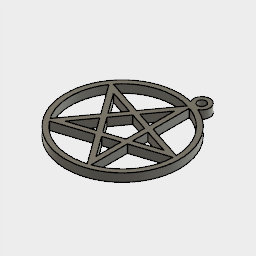
FPROJ_9_LIUYH (Autodesk Fusion 360 design; units mm, degrees)
Autodesk Fusion 360 part; units mm, degrees
sketch "草图1" plane through (0, 0, 0) normal (0, 1, 0) x (1, 0, 0)
  circle A0 centre (-5, 0) radius 34.7082
  arc A1 (-31.2161, 17.8361) -> (-30.0644, 19.4213) centre (-5, 0) ccw
  circle A2 centre (-65, 20) radius 2.5
  circle A3 centre (-65, 20) radius 4
  line L0 (-18.2574, 0) -> (-31.2161, -17.8361)
  line L1 (3.862, -30.4446) -> (-16.4033, -2.552)
  line L2 (-18.2574, 0) -> (-31.2161, 17.8361)
  line L3 (-16.4033, -2.552) -> (-25.2254, -14.6946)
  line L4 (2.7254, -23.7764) -> (-14.5492, 0)
  line L5 (-16.4033, 2.552) -> (-25.2254, 14.6946)
  line L6 (-25.2254, 14.6946) -> (-10.9508, 10.0565)
  line L7 (3.862, 30.4446) -> (-9.0967, 12.6085)
  line L8 (-10.9508, 10.0565) -> (-16.4033, 2.552)
  line L9 (-30.0644, 19.4213) -> (-9.0967, 12.6085)
  line L10 (2.7254, 23.7764) -> (-6.0967, 11.6337)
  line L11 (-7.9508, 9.0818) -> (-14.5492, 0)
  line L12 (-10.9508, -10.0565) -> (-25.2254, -14.6946)
  line L13 (-9.0967, -12.6085) -> (-30.0644, -19.4213)
  line L14 (20, 0) -> (5.7254, -4.6381)
  line L15 (2.7254, -5.6128) -> (-7.9508, -9.0818)
  line L16 (26.6931, -0.9797) -> (5.7254, -7.7925)
  line L17 (2.7254, -8.7672) -> (-6.0967, -11.6337)
  line L18 (-6.0967, 11.6337) -> (2.7254, 8.7672)
  line L19 (5.7254, 7.7925) -> (26.6931, 0.9797)
  line L20 (-7.9508, 9.0818) -> (2.7254, 5.6128)
  line L21 (5.7254, 4.6381) -> (20, 0)
  line L22 (2.7254, 23.7764) -> (2.7254, 8.7672)
  line L23 (5.7254, 29.8392) -> (5.7254, 7.7925)
  line L24 (2.7254, 5.6128) -> (2.7254, -5.6128)
  line L25 (2.7254, -8.7672) -> (2.7254, -23.7764)
  line L26 (5.7254, 4.6381) -> (5.7254, -4.6381)
  line L27 (5.7254, -7.7925) -> (5.7254, -29.8392)
  point P0 (-5, 0)
extrude "拉伸1" add sketch "草图1" along normal blind 5 contours A0 makes body 1
sketch "草图2" plane through (0, 0, 0) normal (0, 1, 0) x (1, 0, 0)
  circle A0 centre (60, 10) radius 2.5
  circle A1 centre (60, 10) radius 5
extrude "拉伸2" add sketch "草图2" along normal blind 5 separate body makes body 2
move_face "MoveFace1" by (-50.0242, 0, -33.1903) 1 faces at (64.1387, 5, -9.6274) on bodies 2
move_body "移动1" bodies 2 to x (1, 0, 0) y (0, 1, 0) z (0, 0, 1) at (-53.1283, 0, -26.2657)
combine "合并1" operation add target body 1 tool bodies 2
